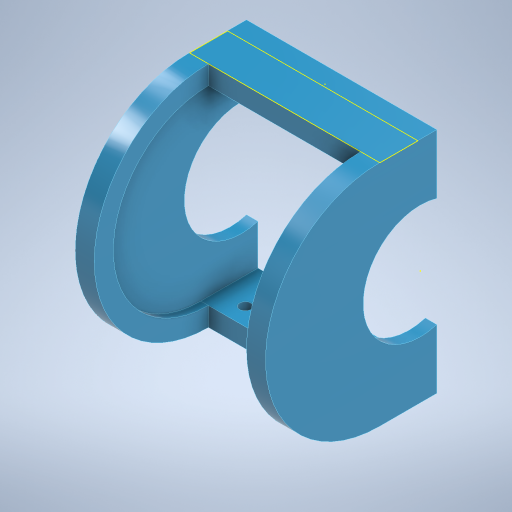
# Autodesk Inventor part: przód2
Saved by Autodesk Inventor 2024 (Build 280153000, 153)
## iProperties
Created: 2025-05-21
Part Number: przód2
Material: Tworzywo sztuczne PET
Document SubType Name: Modeling
Designer: Paweł
Density: 1.541 g/cm^3
Appearance: Ciemnobłękitna
Mass: 29.6632 g
Surface Area: 125.339 cm^2
Volume: 19.2493 cm^3
Author: Paweł
Autodesk Inventor part; units mm, degrees
ref_plane "YZ Plane" through (0, 0, 0) normal (1, 0, 0) x (0, 1, 0)
ref_plane "XZ Plane" through (0, 0, 0) normal (0, 1, 0) x (-1, 0, 0)
sketch "Szkic1" plane through (0, 0, 0) normal (0, 0, 1) x (1, 0, 0)
  line L0 (19.3649, 0) -> (-19.3649, 0)
  line L1 (-19.3649, 0) -> (-103.6215, 0)
  line L2 (-103.6215, 0) -> (-125, 0)
  line L3 (-125, 0) -> (-103.6215, 0)
  line L4 (-103.6215, 0) -> (-19.3649, 0)
  line L5 (-19.3649, 0) -> (19.3649, 0)
  line L6 (19.3649, 0) -> (103.6215, 0)
  line L7 (103.6215, 0) -> (125, 0)
  line L8 (125, 0) -> (103.6215, 0)
  line L9 (103.6215, 0) -> (19.3649, 0)
  line L10 (45, 0) -> (-45, 0)
  line L11 (45, 0) -> (105.3748, 0)
  line L12 (105.3748, 0) -> (130.0712, 0)
  line L13 (130.0712, 0) -> (105.3748, 0)
  line L14 (105.3748, 0) -> (-20.2973, 0)
  line L15 (-20.2973, 0) -> (-105.3748, 0)
  line L16 (-105.3748, 0) -> (-105.3748, 0)
  line L17 (-105.3748, 0) -> (-130.0712, 0)
  line L18 (-130.0712, 0) -> (-105.3748, 0)
  line L19 (-105.3748, 0) -> (-45, 0)
  arc A0 (119.2902, -19.1594) -> (125, 0) centre (90, 0) ccw
  arc A1 (19.3649, -35) -> (103.6215, -25.7743) centre (42.8262, 140.0954) ccw
  arc A2 (103.6215, -25.7743) -> (125, 0) centre (91.4189, 6.1005) ccw
  arc A3 (20.2973, -40.1624) -> (105.3748, -30.457) centre (42.8262, 140.0954) ccw
  arc A4 (105.3748, -30.457) -> (130.0712, 0) centre (91.4189, 6.1005) ccw
  arc A5 (-125, 0) -> (-103.6215, -25.7743) centre (-91.4189, 6.1005) ccw
  arc A6 (-130.0712, 0) -> (-105.3748, -30.457) centre (-91.4189, 6.1005) ccw
  arc A7 (-98.4086, -33.9749) -> (-78.2644, -32.9739) centre (-90, 0) ccw
  arc A8 (-103.6215, -25.7743) -> (-19.3649, -35) centre (-42.8262, 140.0954) ccw
  arc A9 (-19.3649, -35) -> (19.3649, -35) centre (0, 0) ccw
  arc A10 (-20.2973, -40.1624) -> (20.2973, -40.1624) centre (0, 0) ccw
  arc A11 (-105.3748, -30.457) -> (-20.2973, -40.1624) centre (-42.8262, 140.0954) ccw
  line L20 (-105.3748, 0) -> (-20.2973, 0)
  line L21 (19.3649, 0) -> (-19.3649, 0)
  line L22 (130.0712, 0) -> (-130.0712, 0)
  point P0 (0, 0)
  point P1 (-119.2902, -19.1594)
  point P2 (-125, 0)
  point P3 (125, 0)
  dimension "d0" = 70
  dimension "d1" = 70
  dimension "d2" = 250
  dimension "d3" = 90
  constraints: 46 end point, 25 point on circle, 12 centre point, 2 horizontal alignment, 1 coincident, 1 horizontal, 4 other
  measures "d0" diameter of A0
  measures "d1" diameter of A7
  measures "d3" distance of point (0, 0) A7.centre
revolve "Obrót1" add sketch "Szkic1" angle 180 about axis through (130.0712, 0, 0) along (-1, 0, 0) contours L12 A4 A3 A10 A11 A7 A8 A9 A1 A2 | A5 A8 A7 A11 A6 L17
sketch "Szkic2" plane through (0, 0, 0) normal (0, 1, 0) x (-1, 0, 0)
  line L0 (-25, 45) -> (25, 45)
  line L1 (25, 45) -> (25, 15)
  line L2 (25, 15) -> (-25, 15)
  line L3 (-25, 15) -> (-25, 45)
  line L4 (-20.2973, 0) -> (20.2973, 0) projected
  arc A0 (105.3748, 30.457) -> (20.2973, 40.1624) centre (42.8262, -140.0954) ccw projected
  arc A1 (20.2973, 40.1624) -> (-20.2973, 40.1624) centre (0, 0) ccw projected
  point P0 (0, 0)
  point P1 (0, 45)
  point P2 (0, 0)
  point P3 (0, 45)
  dimension "d5" = 50
  dimension "d6" = 30
  constraints: 8 end point, 3 perpendicular, 2 midpoint, 1 coincident, 1 horizontal, 1 point on circle, 1 vertical alignment
  measures "d5" distance of L0.start L0.end
  measures "d6" distance of L0.end L1.end
extrude "Wyciągnięcie proste1" cut sketch "Szkic2" along normal mid plane 91
sketch "Szkic3" plane through (25, 0, 0) normal (-1, 0, 0) x (0, 0, 1)
  point P0 (0, 0)
sketch "Szkic4" plane through (25, 0, 0) normal (-1, 0, 0) x (0, 0, 1)
  arc A0 (15, -37.8222) -> (15, 37.8222) centre (0, 0) ccw projected
  line L0 (15, 37.8222) -> (15, 32.3552) projected
  arc A1 (15, -32.3552) -> (15, 32.3552) centre (0, 0) ccw projected
  line L1 (15, -32.3552) -> (15, -37.8222) projected
  circle A2 centre (10.6631, 0) radius 25
  arc A3 (15, -32.3552) -> (15, 32.3552) centre (0, 0) ccw projected
  circle A4 centre (10.6631, 0) radius 30
  point P0 (0, 0)
  point P1 (35.6631, 0)
  point P2 (22.7682, 27.4494)
  point P3 (22.7682, -27.4494)
  point P4 (35.6631, 0)
  dimension "d9" = 50
  dimension "d19" = 60
  constraints: 1 centre point, 1 coincident, 1 point on circle, 3 other
  measures "d19" diameter of A4
extrude "Wyciągnięcie proste2" add sketch "Szkic4" along normal blind 50 contours A4 A1 | A1 A4
sketch "Szkic5" plane through (25, 0, 10.6631) normal (1, 0, 0) x (0, 0, -1)
  arc A0 (-12.1051, -27.4494) -> (-12.1051, 27.4494) centre (0, 0) ccw projected
  circle A1 centre (0, 0) radius 25 projected
  line L0 (0, 25) -> (0, 30)
  line L1 (0, -25) -> (0, -30)
  point P0 (10.6631, 0)
  point P1 (-12.0349, 27.5074)
  point P2 (-12.0349, -27.5074)
  point P3 (-25, 0)
  constraints: 4 end point, 4 point on circle, 2 vertical
extrude "Wyciągnięcie proste3" cut sketch "Szkic5" against normal blind 50 contours L1 A1 L0 A0
ref_plane "Płaszczyzna konstrukcyjna1" through (0, 0, 0) normal (1, 0, 0) x (0, 0, -1)
sketch "Szkic7" plane through (0, 0, 0) normal (1, 0, 0) x (0, 0, -1)
  arc A0 (-10.6631, 25) -> (-35.6631, 0) centre (-10.6631, 0) ccw projected
  circle A1 centre (-10.6631, 0) radius 25
  circle A2 centre (-10.6631, 0) radius 30
  point P0 (0, 0)
  point P1 (-35.6631, 0)
  dimension "d16" = 5
  constraints: 2 centre point, 1 coincident
  measures "d16" radial gap between concentric circles of A1 A2
extrude "Wyciągnięcie proste4" cut sketch "Szkic7" along normal mid plane 40
sketch "Szkic8" plane through (0, 0, 0) normal (1, 0, 0) x (0, 0, -1)
  point P0 (0, 0)
sketch "Szkic9" plane through (-25, -30, 10.6631) normal (0, 0, -1) x (-1, 0, 0)
  line L0 (-5, 5) -> (-5, 0) projected
  line L1 (0, 0) -> (-5, 0) projected
  line L2 (0, 5) -> (0, 0) projected
  line L3 (-5, 5) -> (0, 5) projected
  line L4 (-45, 0) -> (-45, 5) projected
  line L5 (-50, 5) -> (-45, 5) projected
  line L6 (-50, 0) -> (-50, 5) projected
  line L7 (-45, 0) -> (-50, 0) projected
  line L8 (-5, 60) -> (-5, 55) projected
  line L9 (0, 55) -> (-5, 55) projected
  line L10 (0, 60) -> (0, 55) projected
  line L11 (-5, 60) -> (0, 60) projected
  line L12 (-45, 55) -> (-45, 60) projected
  line L13 (-50, 60) -> (-45, 60) projected
  line L14 (-50, 55) -> (-50, 60) projected
  line L15 (-45, 55) -> (-50, 55) projected
  line L16 (0, 55) -> (-50, 55)
  line L17 (-50, 60) -> (0, 60)
  line L18 (0, 0) -> (0, 5)
  line L19 (-50, 5) -> (-50, 0)
  line L20 (0, 5) -> (-50, 5)
  line L21 (0, 0) -> (-50, 0)
  point P0 (-25, 30)
  constraints: 12 end point, 6 collinear
extrude "Wyciągnięcie proste5" add sketch "Szkic9" along normal blind 10
sketch "Szkic10" plane through (-20, 30, 10.6631) normal (0, 1, 0) x (1, 0, 0)
  line L0 (0, 0) -> (-5, 0) projected
  line L1 (0, 0) -> (40, 0) projected
  line L2 (45, 0) -> (40, 0) projected
  line L3 (45, 0) -> (45, 10) projected
  line L4 (-5, 10) -> (45, 10) projected
  line L5 (-5, 0) -> (-5, 10) projected
  point P0 (20, 10.6631)
sketch "Szkic15" plane through (-25, -30, 0.6631) normal (0, 0, -1) x (-1, 0, 0)
  line L0 (-50, 60) -> (-50, 55) projected
  line L1 (-50, 60) -> (-0.0556, 60)
  line L2 (-0.0556, 60) -> (-0.0556, 70)
  line L3 (-0.0556, 70) -> (-50, 70)
  line L4 (-50, 70) -> (-50, 60)
  line L5 (0, 55) -> (0, 60) projected
  arc A0 (-5.6351, 65) -> (-44.3649, 65) centre (-25, 30) ccw projected
  point P0 (-25, 30)
  point P1 (-25.0278, 70)
  point P2 (-25, 70)
  constraints: 8 end point, 2 parallel, 1 horizontal, 1 horizontal alignment, 1 midpoint, 1 perpendicular, 1 point on circle
extrude "Wyciągnięcie proste6" add sketch "Szkic15" against normal blind 3
sketch "Szkic18" plane through (-20, -25, 10.6631) normal (0, 1, 0) x (1, 0, 0)
  line L0 (0, 0) -> (-5, 0) projected
  line L1 (0, 0) -> (40, 0) projected
  line L2 (45, 0) -> (40, 0) projected
  line L3 (45, 0) -> (45, 10) projected
  line L4 (-5, 10) -> (45, 10) projected
  line L5 (-5, 0) -> (-5, 10) projected
  point P0 (20, 10.6631)
extrude "Wyciągnięcie proste9" add sketch "Szkic18" against normal blind 13.5
sketch "Szkic19" plane through (0, 0, 0) normal (0, 0, -1) x (-1, 0, 0)
  arc A0 (-130.0712, 0) -> (-105.3748, -30.457) centre (-91.4189, 6.1005) ccw projected
  arc A1 (-105.3748, -30.457) -> (-20.2973, -40.1624) centre (-42.8262, 140.0954) ccw projected
  arc A2 (-20.2973, -40.1624) -> (20.2973, -40.1624) centre (0, 0) ccw projected
  arc A3 (20.2973, -40.1624) -> (105.3748, -30.457) centre (42.8262, 140.0954) ccw projected
  arc A4 (105.3748, -30.457) -> (130.0712, 0) centre (91.4189, 6.1005) ccw projected
  arc A5 (130.0712, 0) -> (105.3748, 30.457) centre (91.4189, -6.1005) ccw projected
  arc A6 (105.3748, 30.457) -> (20.2973, 40.1624) centre (42.8262, -140.0954) ccw projected
  arc A7 (20.2973, 40.1624) -> (-20.2973, 40.1624) centre (0, 0) ccw projected
  arc A8 (-20.2973, 40.1624) -> (-105.3748, 30.457) centre (-42.8262, -140.0954) ccw projected
  arc A9 (-105.3748, 30.457) -> (-130.0712, 0) centre (-91.4189, -6.1005) ccw projected
  arc A10 (-103.6215, 25.7743) -> (-125, 0) centre (-91.4189, -6.1005) ccw projected
  arc A11 (-19.3649, 35) -> (-103.6215, 25.7743) centre (-42.8262, -140.0954) ccw projected
  arc A12 (19.3649, 35) -> (-19.3649, 35) centre (0, 0) ccw projected
  arc A13 (103.6215, 25.7743) -> (19.3649, 35) centre (42.8262, -140.0954) ccw projected
  arc A14 (125, 0) -> (103.6215, 25.7743) centre (91.4189, -6.1005) ccw projected
  arc A15 (103.6215, -25.7743) -> (125, 0) centre (91.4189, 6.1005) ccw projected
  arc A16 (19.3649, -35) -> (103.6215, -25.7743) centre (42.8262, 140.0954) ccw projected
  arc A17 (-19.3649, -35) -> (19.3649, -35) centre (0, 0) ccw projected
  arc A18 (-103.6215, -25.7743) -> (-19.3649, -35) centre (-42.8262, 140.0954) ccw projected
  arc A19 (-125, 0) -> (-103.6215, -25.7743) centre (-91.4189, 6.1005) ccw projected
  line L0 (-130.0712, 0) -> (130.0712, 0)
  line L1 (-25, 34.6933) -> (-25, -34.6933) projected
  line L2 (-25, 34.6933) -> (-25, 40.6881)
  line L3 (-25, -34.6933) -> (-25, -40.6881)
  line L4 (25, -27.4494) -> (25, 27.4494) projected
  line L5 (25, 27.4494) -> (25, 40.6881)
  line L6 (25, -27.4494) -> (25, -40.6881)
  point P0 (0, 0)
  point P1 (25, 35.6631)
  point P2 (125, 0)
  point P3 (-125, 0)
  point P4 (-25, 35.6631)
  point P5 (-25, 37.8222)
  point P6 (-25, -37.8222)
  constraints: 10 end point, 4 point on circle, 3 vertical, 1 horizontal
revolve "Obrót4" cut sketch "Szkic19" angle 360 about axis through (130.0712, 0, 0) along (-1, 0, 0) contours A9 A8 L2 A11 A10 L0 | A14 A13 L5 A6 A5 L0
sketch "Szkic20" plane through (0, 0, 0) normal (0, 0, -1) x (-1, 0, 0)
  line L0 (25, -40.6881) -> (25, -35.6631) projected
  arc A0 (25, 40.6881) -> (20.2973, 40.1624) centre (42.8262, -140.0954) ccw projected
  arc A1 (20.2973, 40.1624) -> (-20.2973, 40.1624) centre (0, 0) ccw projected
  arc A2 (-20.2973, 40.1624) -> (-25, 40.6881) centre (-42.8262, -140.0954) ccw projected
  line L1 (-25, 40.6881) -> (-25, 35.6631) projected
  arc A3 (-19.3649, 35) -> (-25, 35.6631) centre (-42.8262, -140.0954) ccw projected
  arc A4 (19.3649, 35) -> (-19.3649, 35) centre (0, 0) ccw projected
  arc A5 (25, 35.6631) -> (19.3649, 35) centre (42.8262, -140.0954) ccw projected
  line L2 (25, -27.4494) -> (25, 27.4494) projected
  line L3 (25, 0) -> (-25, 0)
  arc A6 (19.3649, -35) -> (25, -35.6631) centre (42.8262, 140.0954) ccw projected
  arc A7 (-19.3649, -35) -> (19.3649, -35) centre (0, 0) ccw projected
  arc A8 (-25, -35.6631) -> (-19.3649, -35) centre (-42.8262, 140.0954) ccw projected
  line L4 (-25, -35.6631) -> (-25, -40.6881) projected
  arc A9 (-25, -40.6881) -> (-20.2973, -40.1624) centre (-42.8262, 140.0954) ccw projected
  arc A10 (-20.2973, -40.1624) -> (20.2973, -40.1624) centre (0, 0) ccw projected
  arc A11 (20.2973, -40.1624) -> (25, -40.6881) centre (42.8262, 140.0954) ccw projected
  line L5 (25, 35.6631) -> (25, 40.6881) projected
  point P0 (0, 0)
  point P1 (25, 30)
  point P2 (25, -30)
  constraints: 2 end point, 1 horizontal, 1 midpoint
revolve "Obrót5" cut sketch "Szkic20" angle 30 about axis through (-25, 0, 0) along (1, 0, 0) contours L5 A5 A4 A3 L1 A2 A1 A0
sketch "Szkic23" plane through (0, 0, 0) normal (0, 0, -1) x (-1, 0, 0)
  line L0 (25, -40.6881) -> (25, -35.6631) projected
  arc A0 (19.3649, -35) -> (25, -35.6631) centre (42.8262, 140.0954) ccw projected
  arc A1 (-19.3649, -35) -> (19.3649, -35) centre (0, 0) ccw projected
  arc A2 (-25, -35.6631) -> (-19.3649, -35) centre (-42.8262, 140.0954) ccw projected
  line L1 (-25, -35.6631) -> (-25, -40.6881) projected
  arc A3 (-25, -40.6881) -> (-20.2973, -40.1624) centre (-42.8262, 140.0954) ccw projected
  arc A4 (-20.2973, -40.1624) -> (20.2973, -40.1624) centre (0, 0) ccw projected
  arc A5 (20.2973, -40.1624) -> (25, -40.6881) centre (42.8262, 140.0954) ccw projected
  line L2 (0, 0) -> (-25.9666, 0)
  point P0 (0, 0)
  constraints: 2 end point, 1 horizontal
revolve "Obrót6" cut sketch "Szkic23" angle 30 about axis through (0, 0, 0) along (-1, 0, 0)
sketch "Szkic24" plane through (25, 0, 0) normal (1, 0, 0) x (0, 0, -1)
  arc A0 (-10.6631, -34.0317) -> (-0.6631, -35.657) centre (0, 0) ccw projected
  line L0 (-0.6631, -25) -> (-0.6631, -35.657) projected
  line L1 (-10.6631, -25) -> (-0.6631, -25) projected
  arc A1 (-10.6631, 25) -> (-10.6631, -25) centre (-10.6631, 0) ccw projected
  line L2 (-10.6631, 25) -> (-0.6631, 25) projected
  line L3 (-0.6631, 35.657) -> (-0.6631, 25) projected
  arc A2 (-0.6631, 35.657) -> (-3.6631, 35.4745) centre (0, 0) ccw projected
  line L4 (-3.6631, 30) -> (-3.6631, 35.4745) projected
  line L5 (-10.6631, 30) -> (-3.6631, 30) projected
  arc A3 (-10.6631, 30) -> (-10.6631, -30) centre (-10.6631, 0) ccw projected
  line L6 (-10.6631, -30) -> (-10.6631, -34.0317) projected
  line L7 (-10.6631, -30) -> (-0.6631, -30)
  line L8 (-10.6631, 30) -> (-10.6631, 45.858)
  line L9 (-10.6631, 45.858) -> (14.375, 45.858)
  line L10 (14.375, 45.858) -> (14.375, -45.1514)
  line L11 (14.375, -45.1514) -> (-20.0352, -45.1514)
  line L12 (-10.6631, -30) -> (-10.6631, -34.0317) projected
  line L13 (-20.0352, -45.1514) -> (-10.6631, -30)
  line L14 (-10.6631, 30) -> (-0.6631, 30)
  line L15 (-10.6631, 25) -> (-0.6631, 25) projected
  line L16 (-0.6631, 25) -> (-10.6631, 25)
  point P0 (0, 0)
  constraints: 16 end point, 4 perpendicular, 3 point on line, 1 horizontal, 1 vertical
extrude "Wyciągnięcie proste10" cut sketch "Szkic24" against normal blind 61.5 contours L6 L7 L0 A0 | A0 L0 L1 A1 L2 L3 A2 L4 L5 L8 L9 L10 L11 L13 L6 | L4 A2 L3 L14
sketch "Szkic25" plane through (-20, -25, 10.6631) normal (0, 1, 0) x (1, 0, 0)
  circle A0 centre (35, 4.645) radius 1.5
  circle A1 centre (5, 4.645) radius 1.5
  line L0 (45, 0) -> (45, 10) projected
  point P0 (20, 10.6631)
  dimension "d38" = 3
  dimension "d39" = 3
  dimension "d40" = 10
  dimension "d41" = 30
  constraints: 2 centre point, 1 horizontal alignment
  measures "d38" diameter of A0
  measures "d39" diameter of A1
  measures "d40" distance from line of L0 A0.centre
  measures "d41" distance of A1.centre A0.centre
extrude "Wyciągnięcie proste11" cut sketch "Szkic25" against normal blind 61.5
sketch "Szkic26" plane through (-25, -30, 0.6631) normal (0, 0, -1) x (-1, 0, 0)
  point P0 (-25, 30)
sketch "Szkic27" plane through (-25, -30, 0.6631) normal (0, 0, -1) x (-1, 0, 0)
  line L0 (0, 60) -> (-50, 60) projected
  line L1 (-50, 60) -> (-50, 55) projected
  line L2 (-50, 55) -> (0, 55) projected
  line L3 (0, 55) -> (0, 60) projected
  line L4 (-50, 0) -> (0, 0) projected
  line L5 (0, 5) -> (0, 0) projected
  line L6 (0, 5) -> (-50, 5) projected
  line L7 (-50, 5) -> (-50, 0) projected
  point P0 (-25, 30)
extrude "Wyciągnięcie proste12" add sketch "Szkic27" along normal blind 5
sketch "Szkic28" plane through (25, 0, 0) normal (1, 0, 0) x (0, 0, -1)
  line L0 (-10.6631, -30) -> (4.3369, -30) projected
  line L1 (4.3369, -25) -> (4.3369, -30) projected
  line L2 (-10.6631, -25) -> (4.3369, -25) projected
  arc A0 (-10.6631, 25) -> (-10.6631, -25) centre (-10.6631, 0) ccw projected
  line L3 (-10.6631, 25) -> (4.3369, 25) projected
  line L4 (4.3369, 30) -> (4.3369, 25) projected
  line L5 (-10.6631, 30) -> (4.3369, 30) projected
  arc A1 (-10.6631, 30) -> (-10.6631, -30) centre (-10.6631, 0) ccw projected
  line L6 (4.3369, 25) -> (4.3369, -25)
  point P0 (0, 0)
  constraints: 2 end point, 1 collinear
extrude "Wyciągnięcie proste13" add sketch "Szkic28" against normal blind 3 contours L2 A0 L3 L6
sketch "Szkic29" plane through (-25, 0, 0) normal (-1, 0, 0) x (0, 0, 1)
  line L0 (10.6631, -25) -> (-4.3369, -25) projected
  arc A0 (10.6631, -25) -> (10.6631, 25) centre (10.6631, 0) ccw projected
  line L1 (-4.3369, 25) -> (10.6631, 25) projected
  line L2 (-4.3369, 25) -> (-4.3369, -25) projected
  point P0 (0, 0)
extrude "Wyciągnięcie proste14" add sketch "Szkic29" against normal blind 3
sketch "Szkic30" plane through (25, 0, 0) normal (1, 0, 0) x (0, 0, -1)
  circle A0 centre (0, 0) radius 15
  dimension "d50" = 30
  constraints: 1 centre point, 1 coincident
  measures "d50" diameter of A0
extrude "Wyciągnięcie proste15" cut sketch "Szkic30" against normal blind 71
